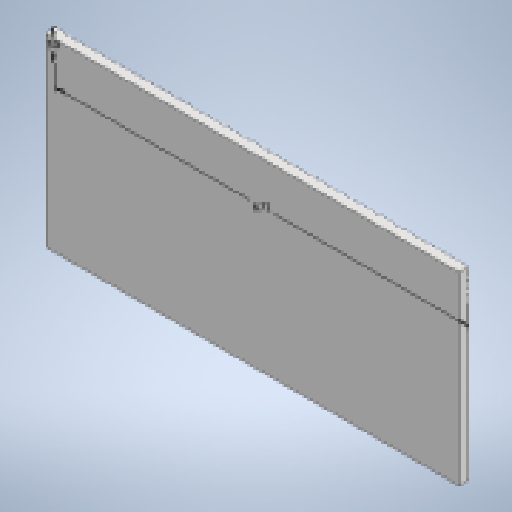
# Autodesk Inventor part: стенка
Saved by Autodesk Inventor 2023.1 (Build 271208000, 208)
## iProperties
Created: 2025-12-01
Part Number: стенка
Material: Типовые
Document SubType Name: Modeling
Designer: DELL
Density: 1 g/cm^3
Appearance: По умолчанию
Author: DELL
Autodesk Inventor part; units mm, degrees
ref_plane "YZ Plane" through (0, 0, 0) normal (1, 0, 0) x (0, 1, 0)
ref_plane "XZ Plane" through (0, 0, 0) normal (0, 1, 0) x (-1, 0, 0)
ref_plane "XY Plane" through (0, 0, 0) normal (0, 0, 1) x (1, 0, 0)
sketch "Эскиз1" plane through (0, 0, 0) normal (0, 0, 1) x (1, 0, 0)
  line L0 (-335.5, 0) -> (335.5, 0)
  line L1 (335.5, 0) -> (335.5, 300)
  line L2 (335.5, 300) -> (-335.5, 300)
  line L3 (-335.5, 300) -> (-335.5, 0)
  point P0 (0, 0)
  point P1 (0, 0)
  dimension "d0" = 671
  dimension "d1" = 300
  constraints: 8 end point, 2 parallel, 1 coincident, 1 horizontal, 1 midpoint, 1 perpendicular
  measures "d0" distance of L2.end L1.end
  measures "d1" distance of L2.end L0.start
extrude "Выдавливание1" add sketch "Эскиз1" along normal blind 16
sketch "Эскиз2" plane through (0, 0, 0) normal (0, 0, -1) x (-1, 0, 0)
  line L0 (-335.5, 300) -> (335.5, 300) construction
  line L1 (335.5, 300) -> (335.5, 250) construction
  line L2 (335.5, 250) -> (-335.5, 250) construction
  line L3 (-335.5, 250) -> (-335.5, 300) construction
  point P0 (0, 0)
  dimension "d4" = 671
  dimension "d5" = 50
  constraints: 8 end point, 2 parallel, 1 horizontal, 1 perpendicular
  measures "d4" distance of L1.end L2.end
  measures "d5" distance of L0.end L1.end
